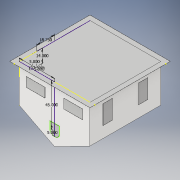
# Autodesk Inventor part: Parthouer
Saved by Autodesk Inventor 2018 (Build 220112000, 112)
## iProperties
Created: 2018-05-30
Part Number: Parthouer
Material: Generic
Document SubType Name: Modeling
Designer: 3400746
Density: 1 g/cm^3
Appearance: Default
Author: 3400746
Autodesk Inventor part; units mm, degrees
ref_plane "YZ Plane" through (0, 0, 0) normal (1, 0, 0) x (0, 1, 0)
ref_plane "XZ Plane" through (0, 0, 0) normal (0, 1, 0) x (-1, 0, 0)
ref_plane "XY Plane" through (0, 0, 0) normal (0, 0, 1) x (1, 0, 0)
sketch "Sketch2" plane through (0, 0, 0) normal (0, 1, 0) x (-1, 0, 0)
  line L0 (0, 0) -> (2159, 0)
  line L1 (2159, 0) -> (2159, -2159)
  line L2 (2159, -2159) -> (0, -2159)
  line L3 (0, -2159) -> (0, 0)
  dimension "d3" = 2159
  dimension "d4" = 2159
  dimension "d5" = 2159
  dimension "d6" = 2159
  constraints: 8 end point, 2 perpendicular, 1 horizontal
  measures "d3" distance of L0.start L0.end
  measures "d4" distance of L0.end L1.end
  measures "d5" distance of L1.end L2.end
  measures "d6" distance of L2.end L0.start
sketch "Sketch4" plane through (0, 0, 0) normal (0, 1, 0) x (-1, 0, 0)
  line L0 (0, 0) -> (0, -127)
  line L1 (2032, -127) -> (2032, -2032)
  line L2 (2032, -127) -> (127, -127)
  line L3 (127, -127) -> (127, -2032)
  line L4 (2032, -2032) -> (127, -2032)
  dimension "d16" = 127
  dimension "d17" = 2032
  dimension "d18" = 1905
  dimension "d20" = 1905
  dimension "d21" = 1905
  constraints: 10 end point, 3 vertical, 1 horizontal
  measures "d16" distance of L0.start L0.end
  measures "d17" distance of L0.end L1.start
  measures "d18" distance of L1.start L1.end
  measures "d20" distance of L1.start L2.end
  measures "d21" distance of L2.end L3.end
extrude "Extrusion3" add sketch "Sketch4" against normal blind 1016
sketch "Sketch5" plane through (-127, 0, -2032) normal (0, 0, -1) x (-1, 0, 0)
  point P0 (-127, 0)
sketch "Sketch6" plane through (-2032, 0, -2032) normal (-1, 0, 0) x (0, 0, 1)
  line L0 (0, 0) -> (952.5, 0)
  line L1 (1905, 0) -> (0, 0) projected
  line L2 (952.5, 0) -> (952.5, -1016)
  line L3 (1905, -1016) -> (0, -1016) projected
  line L4 (952.5, 0) -> (1428.75, 0)
  line L5 (1428.75, 0) -> (1428.75, -355.6)
  line L6 (744.6615, 0) -> (744.6615, -508)
  line L7 (744.6615, -508) -> (216.1341, -508)
  line L8 (216.1341, -508) -> (216.1341, 0)
  line L9 (1428.75, -355.6) -> (1301.75, -355.6)
  line L10 (1301.75, -355.6) -> (1301.75, 0)
  line L11 (1428.75, -355.6) -> (1555.75, -355.6)
  line L12 (1555.75, -355.6) -> (1555.75, 0)
  point P0 (2032, 0)
  dimension "d24" = 476.25
  dimension "d25" = 355.6
  dimension "d26" = 127
  dimension "d27" = 127
  constraints: 22 end point, 5 point on line, 3 horizontal, 3 perpendicular, 2 midpoint, 2 vertical
  measures "d24" distance of L0.end L4.end
  measures "d25" distance of L4.end L5.end
  measures "d26" distance of L5.end L9.end
  measures "d27" distance of L5.end L11.end
extrude "Extrusion4" add sketch "Sketch6" along normal blind 2.54 contours L1 L5 L9 L10 | L1 L12 L11 L5
extrude "Extrusion5" add sketch "Sketch6" along normal blind 2.54 contours L0 L6 L7 L8
sketch "Sketch7" plane through (-127, 0, -2032) normal (0, 0, -1) x (-1, 0, 0)
  line L0 (1905, 0) -> (1905, -1016) projected
  line L1 (1905, 0) -> (0, 0) projected
  line L2 (952.5, 0) -> (952.5, -2181.7197)
  line L3 (1905, -1016) -> (952.5, -1505.9188)
  line L4 (1905, -1016) -> (0, -1016) projected
  line L5 (952.5, -1505.9188) -> (0, -1016)
  line L6 (1905, -1016) -> (0, -1016)
  point P0 (-127, 0)
  constraints: 8 end point, 1 collinear, 1 midpoint, 1 point on line, 1 vertical
extrude "Extrusion6" add sketch "Sketch7" against normal blind 1905 contours L3 L2 L4 | L5 L4 L2
extrude "Extrusion7" add sketch "Sketch2" along normal blind 2.54
sketch "Sketch9" plane through (-2032, 0, -127) normal (0, 0, 1) x (1, 0, 0)
  line L0 (-127, 2.54) -> (2032, 2.54) projected
  line L1 (-2.2534, 2.54) -> (950.2466, 2.54)
  line L2 (950.2466, 2.54) -> (950.2466, -864.9635)
  line L3 (950.2466, 2.54) -> (950.2466, -251.46)
  line L4 (950.2466, -251.46) -> (950.2466, -505.46)
  line L5 (696.2466, -251.46) -> (696.2466, -505.46)
  line L6 (696.2466, -505.46) -> (188.2466, -505.46)
  line L7 (188.2466, -505.46) -> (188.2466, -251.46)
  line L8 (188.2466, -251.46) -> (696.2466, -251.46)
  line L9 (1204.2466, -251.46) -> (1204.2466, -505.46)
  line L10 (1204.2466, -505.46) -> (1712.2466, -505.46)
  line L11 (1712.2466, -505.46) -> (1712.2466, -251.46)
  line L12 (1712.2466, -251.46) -> (1204.2466, -251.46)
  point P0 (2032, 0)
  dimension "d40" = 952.5
  dimension "d41" = 254
  dimension "d46" = 254
  dimension "d47" = 508
  dimension "d48" = 254
  dimension "d49" = 254
  dimension "d51" = 508
  dimension "d52" = 254
  constraints: 24 end point, 5 vertical, 4 point on line, 1 collinear, 1 horizontal, 1 perpendicular
  measures "d40" distance of L1.start L1.end
  measures "d41" distance of L1.end L3.end
  measures "d46" distance of L5.start L5.end
  measures "d47" distance of L5.end L6.end
  measures "d48" distance of L6.end L7.end
  measures "d49" distance of L3.end L9.start
  measures "d51" distance of L9.end L10.end
  measures "d52" distance of L10.end L11.end
extrude "Extrusion8" add sketch "Sketch9" along normal blind 2.54
sketch "Sketch10" plane through (-2032, 0, -127) normal (0, 0, 1) x (1, 0, 0)
  line L0 (0, 0) -> (0, -355.6) projected
  line L1 (0, 0) -> (952.5, 0)
  line L2 (1905, 0) -> (0, 0) projected
  line L3 (952.5, 0) -> (952.5, -1143)
  line L4 (952.5, -1143) -> (952.5, -1270)
  line L5 (825.5, -965.2) -> (1079.5, -965.2)
  arc A0 (825.5, -1181.1) -> (1079.5, -1181.1) centre (952.5, -1134.8357) ccw
  line L6 (1079.5, -1181.1) -> (1079.5, -965.2)
  line L7 (825.5, -1181.1) -> (825.5, -965.2)
  point P0 (2032, 0)
  dimension "d55" = 952.5
  dimension "d56" = 1143
  dimension "d58" = 127
  constraints: 12 end point, 3 point on circle, 2 vertical, 1 centre point, 1 horizontal, 1 midpoint
  measures "d55" distance of L0.start L1.end
  measures "d56" distance of L1.end L3.end
  measures "d58" distance of L3.end L4.end
extrude "Extrusion9" add sketch "Sketch10" along normal blind 2.54
sketch "Sketch11" plane through (-127, -1016, -127) normal (1, 0, 0) x (0, 0, -1)
  line L0 (0, 1016) -> (349.25, 1016) projected
  line L1 (0, 1016) -> (476.25, 1016)
  line L2 (476.25, 1016) -> (952.5, 1016)
  line L3 (952.5, 1016) -> (1428.7432, 1018.54)
  line L4 (2032, 1018.54) -> (-127, 1018.54) projected
  line L5 (1905, 1016) -> (1905, 0) projected
  line L6 (1428.7432, 1018.54) -> (1905, 1016)
  line L7 (1428.7432, 1018.54) -> (1428.7432, 0)
  line L8 (952.5, 1016) -> (952.5, 0)
  line L9 (476.25, 1016) -> (476.25, 0)
  line L10 (1428.7432, 1018.54) -> (1428.7432, 815.34)
  line L11 (1428.7432, 815.34) -> (1555.7432, 815.34)
  line L12 (1555.7432, 815.34) -> (1555.7432, 307.34)
  line L13 (1555.7432, 307.34) -> (1301.7432, 307.34)
  line L14 (1301.7432, 307.34) -> (1301.7432, 815.34)
  line L15 (1428.7432, 815.34) -> (1301.7432, 815.34)
  line L16 (476.25, 1013.46) -> (476.25, 810.26)
  line L17 (476.25, 810.26) -> (603.25, 810.26)
  line L18 (603.25, 810.26) -> (603.25, 302.26)
  line L19 (603.25, 302.26) -> (349.25, 302.26)
  line L20 (476.25, 810.26) -> (349.25, 810.26)
  line L21 (-127, 1016) -> (-127, 1018.54) projected
  line L22 (349.25, 302.26) -> (349.25, 810.26)
  dimension "d66" = 476.25
  dimension "d67" = 476.25
  dimension "d68" = 476.25
  dimension "d70" = 127
  dimension "d74" = 254
  dimension "d75" = 508
  dimension "d76" = 203.2
  dimension "d77" = 127
  dimension "d78" = 508
  dimension "d79" = 254
  dimension "d80" = 127
  constraints: 38 end point, 5 point on line, 4 horizontal, 4 perpendicular, 4 vertical, 1 collinear
  measures "d66" distance of L0.start L1.end
  measures "d67" distance of L1.end L2.end
  measures "d68" distance of L2.end L3.end
  measures "d70" distance of L10.end L11.end
  measures "d74" distance of L12.end L13.end
  measures "d75" distance of L13.end L14.end
  measures "d76" distance of L16.start L16.end
  measures "d77" distance of L16.end L17.end
  measures "d78" distance of L17.end L18.end
  measures "d79" distance of L18.end L19.end
  measures "d80" distance of L16.end L20.end
extrude "Extrusion10" add sketch "Sketch11" along normal blind 2.54
sketch "Sketch13" plane through (-127, 0, -2032) normal (0, 0, -1) x (-1, 0, 0)
  line L0 (1905, 0) -> (952.5, 0)
  line L1 (1905, 0) -> (0, 0) projected
  line L2 (700.7534, -251.46) -> (700.7534, -505.46) projected
  line L3 (700.7534, -251.46) -> (700.7534, -505.46)
  line L4 (700.7534, -505.46) -> (192.7534, -505.46)
  line L5 (192.7534, -505.46) -> (192.7534, -251.46)
  line L6 (700.7534, -251.46) -> (192.7534, -251.46)
  line L7 (1206.5, -254) -> (1206.5, -508)
  line L8 (1206.5, -508) -> (1714.5, -508)
  line L9 (1714.5, -508) -> (1714.5, -254)
  line L10 (1714.5, -254) -> (1206.5, -254)
  line L11 (952.5, 0) -> (952.5, -1270)
  line L12 (952.5, -1270) -> (1079.5, -1270)
  line L13 (1079.5, -1270) -> (1079.5, -977.9)
  line L14 (952.5, -1270) -> (825.5, -1270)
  line L15 (825.5, -1270) -> (825.5, -977.9)
  line L16 (1079.5, -977.9) -> (825.5, -977.9)
  line L17 (1079.5, -1270) -> (1079.5, -1206.5)
  line L18 (825.5, -1270) -> (825.5, -1206.5)
  arc A0 (825.5, -1206.5) -> (1079.5, -1206.5) centre (952.5, -1111.25) ccw
  point P0 (-127, 0)
  dimension "d83" = 952.5
  dimension "d87" = 508
  dimension "d88" = 254
  dimension "d89" = 254
  dimension "d90" = 508
  dimension "d91" = 254
  dimension "d92" = 1270
  dimension "d93" = 127
  dimension "d94" = 292.1
  dimension "d95" = 127
  dimension "d96" = 292.1
  dimension "d98" = 63.5
  dimension "d99" = 63.5
  constraints: 34 end point, 5 vertical, 4 horizontal, 3 point on circle, 2 point on line, 1 centre point, 1 collinear, 1 midpoint, 1 perpendicular
  measures "d83" distance of L0.start L0.end
  measures "d87" distance of L2.end L4.end
  measures "d88" distance of L4.end L5.end
  measures "d89" distance of L7.start L7.end
  measures "d90" distance of L7.end L8.end
  measures "d91" distance of L8.end L9.end
  measures "d92" distance of L0.end L11.end
  measures "d93" distance of L11.end L12.end
  measures "d94" distance of L12.end L13.end
  measures "d95" distance of L11.end L14.end
  measures "d96" distance of L14.end L15.end
  measures "d98" distance of L12.end L17.end
  measures "d99" distance of L14.end L18.end
extrude "Extrusion11" add sketch "Sketch13" along normal blind 2.54 contours L2 L4 L5 L6 | L10 L9 L8 L7 | L16 L13 A0 L11 | L11 A0 L15 L16
sketch "Sketch14" plane through (-2032, -355.6, -730.25) normal (-1, 0, 0) x (0, 0, 1)
  line L0 (-1301.75, 355.6) -> (603.25, 355.6) projected
  line L1 (-349.25, 355.6) -> (-349.25, -406.4)
  line L2 (0, 0) -> (254, 0) projected
  line L3 (0, -177.8) -> (-349.25, -177.8)
  line L4 (0, -177.8) -> (0, -406.4)
  line L5 (0, -177.8) -> (254, -177.8)
  line L6 (254, -177.8) -> (254, -406.4)
  line L7 (127, -177.8) -> (127, -469.9)
  arc A0 (0, -406.4) -> (254, -406.4) centre (127, -311.15) ccw
  point P0 (730.25, 355.6)
  dimension "d102" = 762
  dimension "d109" = 228.6
  dimension "d110" = 254
  dimension "d111" = 228.6
  dimension "d112" = 292.1
  constraints: 12 end point, 4 vertical, 3 point on circle, 2 midpoint, 1 centre point, 1 horizontal, 1 perpendicular, 1 point on line
  measures "d102" distance of L1.start L1.end
  measures "d109" distance of L3.start L4.end
  measures "d110" distance of L3.start L5.end
  measures "d111" distance of L5.end L6.end
  measures "d112" distance of L7.start L7.end
extrude "Extrusion12" add sketch "Sketch14" along normal blind 2.54
body "Solid2"
